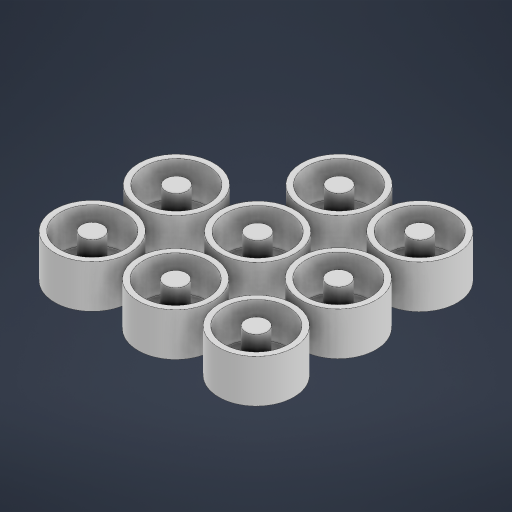
# Autodesk Inventor part: BUTTON
Saved by Autodesk Inventor 2024 (Build 280153000, 153)
## iProperties
Created: 2025-06-23
Part Number: BUTTON
Material: Generic
Document SubType Name: Modeling
Designer: ASUS
Density: 1 g/cm^3
Appearance: Default
Author: ASUS
Autodesk Inventor part; units mm, degrees
ref_plane "YZ Plane" through (0, 0, 0) normal (1, 0, 0) x (0, 1, 0)
ref_plane "XZ Plane" through (0, 0, 0) normal (0, 1, 0) x (-1, 0, 0)
ref_plane "XY Plane" through (0, 0, 0) normal (0, 0, 1) x (1, 0, 0)
sketch "Sketch1" plane through (0, 0, 0) normal (0, 1, 0) x (-1, 0, 0)
  circle A0 centre (0, 0) radius 7
  circle A1 centre (15.1273, 0) radius 7
  circle A2 centre (-15.0261, 0) radius 7
  circle A3 centre (0, -15.1556) radius 7
  circle A4 centre (0, 15.2765) radius 7
  circle A5 centre (-15.0261, 15.2765) radius 7
  circle A6 centre (15.5174, 15.2765) radius 7
  circle A7 centre (-15.0261, -15.1556) radius 7
  dimension "d0" = 14
  dimension "d1" = 14
  dimension "d2" = 14
  dimension "d3" = 14
  dimension "d4" = 14
  dimension "d5" = 14
  dimension "d6" = 14
  dimension "d7" = 14
  constraints: 8 centre point, 1 coincident
  measures "d0" diameter of A0
  measures "d1" diameter of A1
  measures "d2" diameter of A2
  measures "d3" diameter of A3
  measures "d4" diameter of A4
  measures "d5" diameter of A5
  measures "d6" diameter of A6
  measures "d7" diameter of A7
extrude "Extrusion1" add sketch "Sketch1" along normal blind 8
sketch "Sketch17" plane through (0, 8, -15.1556) normal (0, 1, 0) x (1, 0, 0)
  circle A0 centre (0, 0) radius 6
  circle A1 centre (0, 0) radius 2
  point P0 (0, -15.1556)
  dimension "d70" = 12
  dimension "d71" = 4
  constraints: 2 centre point, 1 coincident
  measures "d70" diameter of A0
  measures "d71" diameter of A1
extrude "Extrusion16" cut sketch "Sketch17" against normal blind 6.5
sketch "Sketch18" plane through (15.0261, 8, -15.1556) normal (0, 1, 0) x (1, 0, 0)
  circle A0 centre (0, 0) radius 6
  circle A1 centre (0, 0) radius 2
  point P0 (-15.0261, -15.1556)
  dimension "d74" = 12
  dimension "d75" = 4
  constraints: 2 centre point, 1 coincident
  measures "d74" diameter of A0
  measures "d75" diameter of A1
extrude "Extrusion17" cut sketch "Sketch18" against normal blind 6.5
sketch "Sketch19" plane through (-15.1273, 8, 0) normal (0, 1, 0) x (1, 0, 0)
  circle A0 centre (0, 0) radius 6
  circle A1 centre (0, 0) radius 2
  point P0 (15.1273, 0)
  dimension "d78" = 12
  dimension "d79" = 4
  constraints: 2 centre point, 1 coincident
  measures "d78" diameter of A0
  measures "d79" diameter of A1
extrude "Extrusion18" cut sketch "Sketch19" against normal blind 6.5
sketch "Sketch20" plane through (0, 8, 0) normal (0, 1, 0) x (1, 0, 0)
  circle A0 centre (0, 0) radius 6
  circle A1 centre (0, 0) radius 2
  dimension "d82" = 12
  dimension "d83" = 4
  constraints: 2 centre point, 2 coincident
  measures "d82" diameter of A0
  measures "d83" diameter of A1
extrude "Extrusion19" cut sketch "Sketch20" against normal blind 6.5
sketch "Sketch21" plane through (15.0261, 8, 0) normal (0, 1, 0) x (1, 0, 0)
  circle A0 centre (0, 0) radius 6
  circle A1 centre (0, 0) radius 2
  point P0 (-15.0261, 0)
  dimension "d86" = 12
  dimension "d87" = 4
  constraints: 2 centre point, 1 coincident
  measures "d86" diameter of A0
  measures "d87" diameter of A1
extrude "Extrusion20" cut sketch "Sketch21" against normal blind 6.5
sketch "Sketch22" plane through (-15.5174, 8, 15.2765) normal (0, 1, 0) x (1, 0, 0)
  circle A0 centre (0, 0) radius 6
  circle A1 centre (0, 0) radius 2
  point P0 (15.5174, 15.2765)
  dimension "d90" = 12
  dimension "d91" = 4
  constraints: 2 centre point, 1 coincident
  measures "d90" diameter of A0
  measures "d91" diameter of A1
extrude "Extrusion21" cut sketch "Sketch22" against normal blind 6.5
sketch "Sketch23" plane through (0, 8, 15.2765) normal (0, 1, 0) x (1, 0, 0)
  circle A0 centre (0, 0) radius 6
  circle A1 centre (0, 0) radius 2
  point P0 (0, 15.2765)
  dimension "d94" = 12
  dimension "d95" = 4
  constraints: 2 centre point, 1 coincident
  measures "d94" diameter of A0
  measures "d95" diameter of A1
extrude "Extrusion22" cut sketch "Sketch23" against normal blind 6.5
sketch "Sketch24" plane through (15.0261, 8, 15.2765) normal (0, 1, 0) x (1, 0, 0)
  circle A0 centre (0, 0) radius 6
  circle A1 centre (0, 0) radius 2
  point P0 (-15.0261, 15.2765)
  dimension "d98" = 12
  dimension "d99" = 4
  constraints: 2 centre point, 1 coincident
  measures "d98" diameter of A0
  measures "d99" diameter of A1
extrude "Extrusion23" cut sketch "Sketch24" against normal blind 6.5
body "Solid1"
